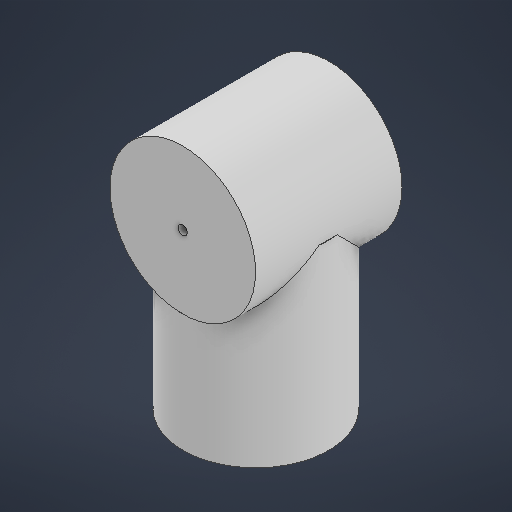
# Autodesk Inventor part: Part6
Saved by Autodesk Inventor 2027.1 (Build 311267000, 267)
## iProperties
Created: 2026-10-02
Part Number: Part6
Material: Generic
Document SubType Name: Modeling
Designer: HP
Density: 1 g/cm^3
Appearance: Default
Author: HP
Autodesk Inventor part; units mm, degrees
ref_plane "YZ Plane" through (0, 0, 0) normal (1, 0, 0) x (0, 1, 0)
ref_plane "XZ Plane" through (0, 0, 0) normal (0, 1, 0) x (-1, 0, 0)
ref_plane "XY Plane" through (0, 0, 0) normal (0, 0, 1) x (1, 0, 0)
sketch "Sketch1" plane through (0, 0, 0) normal (0, 1, 0) x (-1, 0, 0)
  circle A0 centre (0, 0) radius 40
  dimension "d0" = 80
  constraints: 1 centre point, 1 coincident
  measures "d0" diameter of A0
extrude "Extrusion1" add sketch "Sketch1" along normal blind 100
sketch "Sketch2" plane through (0, 100, 0) normal (0, 1, 0) x (1, 0, 0)
  line L0 (-10.8438, 4.9816) -> (0, 4.9816)
  line L1 (0, 4.9816) -> (0, -2.1726)
  line L2 (0, -2.1726) -> (-10.8438, -2.1726)
  line L3 (-10.8438, -2.1726) -> (-10.8438, 4.9816)
  point P0 (0, 0)
  constraints: 8 end point, 2 parallel, 1 horizontal, 1 perpendicular
extrude "Extrusion2" add sketch "Sketch2" along normal blind 10
sketch "Sketch3" plane through (-10.8438, 100, 2.1726) normal (0, 0, 1) x (1, 0, 0)
  line L0 (10.8438, 0) -> (10.8438, 10) projected
  circle A0 centre (10.8438, 5) radius 40
  point P0 (10.8438, -100)
  dimension "d5" = 80
  constraints: 1 centre point, 1 midpoint
  measures "d5" diameter of A0
extrude "Extrusion3" add sketch "Sketch3" along normal blind 38 and the other way blind 42.5
sketch "Sketch4" plane through (-10.8438, 100, 40.1726) normal (0, 0, 1) x (1, 0, 0)
  circle A0 centre (10.8438, 5) radius 2.5527
  line L0 (9.4087, 7.1111) -> (12.2789, 7.1111)
  circle A1 centre (10.8438, 5) radius 40 projected
  point P0 (10.8438, -100)
  dimension "d10" = 5.1054
  dimension "d11" = 2.8702
  constraints: 2 end point, 2 point on circle, 1 centre point, 1 concentric, 1 horizontal
  measures "d10" diameter of A0
  measures "d11" distance of L0.start L0.end
extrude "Extrusion4" cut sketch "Sketch4" against normal blind 22.5044 contours A0 L0 picked at (10.9442, 5.5624)
sketch "Sketch5" plane through (0, 0, 0) normal (0, -1, 0) x (1, 0, 0)
  circle A0 centre (0, 0) radius 2.5527
  line L0 (1.4351, -2.1111) -> (-1.4351, -2.1111)
  dimension "d14" = 5.1054
  dimension "d15" = 2.8702
  constraints: 2 end point, 2 point on circle, 1 centre point, 1 coincident, 1 horizontal
  measures "d14" diameter of A0
  measures "d15" distance of L0.start L0.end
extrude "Extrusion5" cut sketch "Sketch5" against normal blind 10 contours A0 L0 picked at (0.1004, -0.5624)
sketch "Sketch6" plane through (0, 105, -40.3274) normal (0, 0, -1) x (-1, 0, 0)
  line L0 (-21.15, -21.15) -> (21.15, -21.15)
  line L1 (21.15, -21.15) -> (21.15, 21.15)
  line L2 (21.15, 21.15) -> (-21.15, 21.15)
  line L3 (-21.15, 21.15) -> (-21.15, -21.15)
  line L4 (-21.15, -21.15) -> (21.15, 21.15) construction
  line L5 (21.15, -21.15) -> (-21.15, 21.15) construction
  circle A0 centre (0, 0) radius 40 projected
  point P0 (0, -105)
  dimension "d18" = 42.3
  dimension "d19" = 42.3
  dimension "d27" = 21.15
  dimension "d28" = 21.15
  constraints: 12 end point, 2 midpoint, 2 parallel, 1 horizontal, 1 perpendicular
  measures "d18" distance of L0.end L1.end
  measures "d19" distance of L1.end L2.end
  measures "d27" distance from line of A0.centre L3
  measures "d28" distance from line of A0.centre L2
extrude "Extrusion6" cut sketch "Sketch6" against normal blind 22.3 contours L3 L2 L1 L0
sketch "Sketch7" plane through (0, 105, -18.0274) normal (0, 0, -1) x (-1, 0, 0)
  circle A0 centre (0, 0) radius 11.303
  circle A1 centre (0, 0) radius 40 projected
  point P0 (0, -105)
  dimension "d22" = 22.606
  constraints: 1 centre point, 1 concentric
  measures "d22" diameter of A0
extrude "Extrusion7" cut sketch "Sketch7" against normal blind 2.3114 contours A0
sketch "Sketch8" plane through (0, 105, -15.716) normal (0, 0, -1) x (-1, 0, 0)
  circle A0 centre (0, 0) radius 2.5527
  line L0 (2.1111, 1.4351) -> (2.1111, -1.4351)
  circle A1 centre (0, 0) radius 40 projected
  point P0 (0, -105)
  dimension "d25" = 5.1054
  dimension "d26" = 2.8702
  constraints: 2 end point, 2 point on circle, 1 centre point, 1 concentric, 1 vertical
  measures "d25" diameter of A0
  measures "d26" distance of L0.start L0.end
extrude "Extrusion8" cut sketch "Sketch8" against normal blind 60 contours L0 A0 picked at (0.5627, -0.1029)
body "Solid1"
